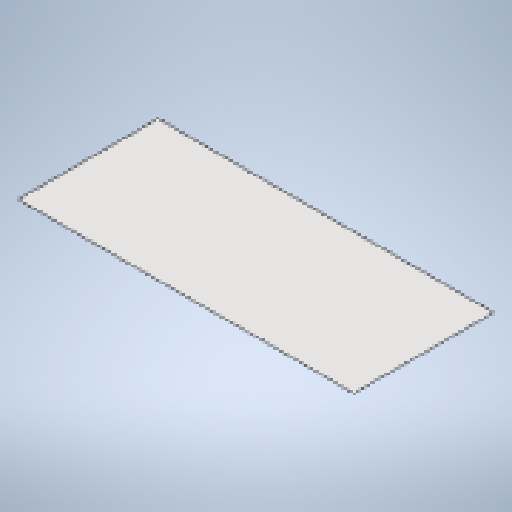
# Autodesk Inventor part: GnG floor sheet 1
Saved by Autodesk Inventor 2025 (Build 290162010, 162A)
## iProperties
Created: 2025-09-20
Part Number: GnG floor sheet 1
Material: Stainless Steel
Document SubType Name: Sheet Metal
Designer: admin
Mass: 360000 g
Surface Area: 300510 cm^2
Volume: 45000 cm^3
Density: 8 g/cm^3
Sheet Metal Rule: AISI304 3mm Die 32
Sheet Metal Width: 0,000 mm
Sheet Metal Length: 0,000 mm
Sheet Metal Area: 0,000 mm^2
Appearance: Default
Author: admin
Autodesk Inventor part; units mm, degrees
ref_plane "YZ Plane" through (0, 0, 0) normal (1, 0, 0) x (0, 1, 0)
ref_plane "XZ Plane" through (0, 0, 0) normal (0, 1, 0) x (-1, 0, 0)
ref_plane "XY Plane" through (0, 0, 0) normal (0, 0, 1) x (1, 0, 0)
sketch "Sketch1" plane through (0, 0, 0) normal (0, 0, 1) x (1, 0, 0)
  line L0 (-3000, -1250) -> (3000, -1250)
  line L1 (3000, -1250) -> (3000, 1250)
  line L2 (3000, 1250) -> (-3000, 1250)
  line L3 (-3000, 1250) -> (-3000, -1250)
  line L4 (-3000, -1250) -> (3000, 1250) construction
  line L5 (3000, -1250) -> (-3000, 1250) construction
  point P0 (0, 0)
  dimension "d0" = 6000
  dimension "d1" = 2500
  measures "d0" distance of L2.end L1.end
  measures "d1" distance of L1.end L0.end
extrude "Plate1" add sketch "Sketch1" along normal blind 3
equation "\"d2\" = Thickness"
equation "\"BendReliefWidth\" = Thickness"
equation "\"BendReliefDepth\" = 0.5 * Thickness"
equation "\"CornerReliefSize\" = 4 * Thickness"
equation "\"MinimumRemnant\" = 2 * Thickness"
equation "\"TransitionRadius\" = BendRadius"
equation "\"JacobiRadiusSize\" = BendRadius"
equation "\"GapSize\" = Thickness"
equation "\"Thickness\" = 3"
equation "\"BendRadius\" = 5"
body "Solid1"
